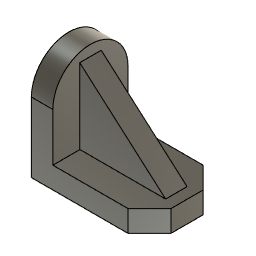
A1 (Autodesk Fusion 360 design; units mm, degrees)
Autodesk Fusion 360 part; units mm, degrees
sketch "Sketch1" plane through (0, 0, 0) normal (0, 0, 1) x (1, 0, 0)
  line L0 (-42, 4) -> (-108, 4)
  line L1 (-108, 4) -> (-108, 46)
  line L2 (-108, 46) -> (-42, 46)
  line L3 (-42, 46) -> (-42, 4)
  line L4 (-42, 4) -> (-108, 46) construction
  line L5 (-108, 4) -> (-42, 46) construction
  point P0 (-75, 25)
  dimension "d1" = 66
  dimension "d2" = 42
  constraint horizontal L0
  constraint perpendicular L0 L1
  constraint parallel L0 L2
  constraint parallel L1 L3
  constraint coincident L4 P0
  constraint coincident L5 P0
  measures "d1" distance of L1.end L2.end
  measures "d2" distance of L0.end L1.end
extrude "Extrude1" add sketch "Sketch1" along normal blind 12 makes body 1
chamfer "Chamfer1" distance 12 angle 45 2 edges at (-42, 4, 6) (-42, 46, 6) on bodies 1
sketch "Sketch2" plane through (0, 0, 12) normal (0, 0, 1) x (-1, 0, 0)
  line L0 (42, -34) -> (54, -46)
  line L1 (54, -46) -> (108, -46)
  line L2 (108, -46) -> (108, -4)
  line L3 (108, -4) -> (54, -4)
  line L4 (54, -4) -> (42, -16)
  line L5 (42, -16) -> (42, -34)
  line L6 (108, -46) -> (96, -46)
  line L7 (96, -46) -> (96, -4)
  line L8 (96, -4) -> (108, -4)
  line L9 (108, -4) -> (108, -46)
  dimension "d6" = 12
  constraint horizontal L6
  constraint vertical L7
  constraint horizontal L8
  constraint vertical L9
  constraint coincident L1.end L2.start
  measures "d6" distance of L1.end L6.end
extrude "Extrude2" add sketch "Sketch2" along normal blind 48 contours L1 L2 L3 L6 L7 L8 L9 bodies 1
fillet "Fillet1" radius 21 2 edges at (-102, 4, 60) (-102, 46, 60) on bodies 1
sketch "Sketch3" plane through (0, 0, 0) normal (0, 1, 0) x (1, 0, 0)
  line L0 (-95.9808, -54.1235, 25) -> (-95.9808, -12.1235, 25)
  line L1 (-95.9808, -12.1235, 25) -> (-47.9808, -12.1235, 25)
  line L2 (-47.9808, -12.1235, 25) -> (-95.9808, -54.1235, 25)
  dimension "d11" = 42
  dimension "d12" = 48
extrude "Extrude3" add sketch "Sketch3" along normal mid plane 12 separate body contours L0 L1 L2 in plane through (0, 25, 0) normal (0, 1, 0) makes body 2
equation "d7 = 60 mm - 12 mm"
equation "d12 = 60 mm - 12 mm"
